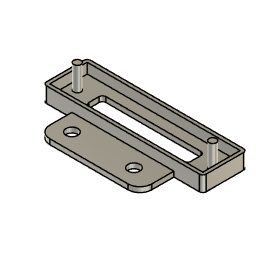
powerdist_ground_mount v2 (Autodesk Fusion 360 design; units mm, degrees)
Autodesk Fusion 360 part; units mm, degrees
sketch "Sketch1" plane through (0, 0, 0) normal (0, 0, 1) x (1, 0, 0)
  line L0 (0, 0) -> (94, 0)
  line L1 (94, 0) -> (94, 26)
  line L2 (94, 26) -> (0, 26)
  line L3 (0, 26) -> (0, 0)
  dimension "d1" = 94
  dimension "d2" = 26
  constraint horizontal L0
  constraint vertical L1
  constraint horizontal L2
  constraint vertical L3
  constraint coincident L0.start L3.end
  measures "d1" distance of L0.start L0.end
  measures "d2" distance of L0.start L2.end
extrude "Extrude1" add sketch "Sketch1" along normal blind 3
extrude "Extrude2" add 1 faces at (31.3333, 17.3333, 3) along direction (0, 0, 1) blind 6 thin wall 2 inside
sketch "Sketch2" plane through (0, 0, 3) normal (0, 0, 1) x (-1, 0, 0)
  line L0 (-92, -24) -> (-2, -24)
  line L1 (-2, -24) -> (-2, -2)
  line L2 (-2, -2) -> (-92, -2)
  line L3 (-92, -2) -> (-92, -24)
  circle A0 centre (-7.15, -13) radius 2.15
  circle A1 centre (-86.85, -13) radius 2.15
  dimension "d8" = 4.3
  dimension "d9" = 4.3
  dimension "d10" = 5.15
  dimension "d11" = 11
  dimension "d12" = 11
  dimension "d13" = 5.15
  measures "d8" diameter of A0
  measures "d9" diameter of A1
  measures "d10" distance of L1 A0.centre
  measures "d11" distance of L2 A0.centre
  measures "d12" distance of L2 A1.centre
  measures "d13" distance of L3 A1.centre
extrude "Extrude3" add sketch "Sketch2" along normal blind 14 contours A0 | A1
fillet "Fillet1" radius 2 4 edges at (94, 0, 4.5) (94, 26, 4.5) (0, 26, 4.5) (0, 0, 4.5)
sketch "Sketch3" plane through (0, 0, 9) normal (0, 0, 1) x (-1, 0, 0)
  line L0 (-2, -24) -> (-92, -24)
  line L1 (-92, -24) -> (-92, -2)
  line L2 (-92, -2) -> (-2, -2)
  line L3 (-2, -2) -> (-2, -24)
  arc A0 (0, -2) -> (-2, 0) centre (-2, -2) ccw
  line L4 (-2, 0) -> (-92, 0)
  arc A1 (-92, 0) -> (-94, -2) centre (-92, -2) ccw
  line L5 (-94, -2) -> (-94, -24)
  arc A2 (-94, -24) -> (-92, -26) centre (-92, -24) ccw
  line L6 (-92, -26) -> (-2, -26)
  arc A3 (-2, -26) -> (0, -24) centre (-2, -24) ccw
  line L7 (0, -24) -> (0, -2)
  line L8 (-77, 13) -> (-77, 0)
  arc A4 (-70, 20) -> (-77, 13) centre (-70, 13) ccw
  circle A5 centre (-63.5, 10) radius 3.5
  line L9 (-24, 20) -> (-70, 20)
  line L10 (-77, 0) -> (-17, 0)
  line L11 (-17, 0) -> (-17, 13)
  circle A6 centre (-27, 10) radius 3.5
  line L12 (-10.5, 0) -> (-76.5, 0)
  arc A7 (-17, 13) -> (-24, 20) centre (-24, 13) ccw
  point P0 (-43.5, 0)
  point P1 (-17, 20)
  dimension "d18" = 20
  dimension "d19" = 60
  dimension "d20" = 7
  dimension "d21" = 7
  dimension "d22" = 10
  dimension "d23" = 7
  constraint coincident L10.end L12
  constraint coincident P1 L11
  constraint coincident P1 L9
  constraint tangent L11 A7
  constraint tangent L9 A7
  constraint tangent A4 L9
  constraint tangent L8 A4
  constraint equal A4 A7
  constraint midpoint L4 L10
  measures "d18" distance of L10.end P1
  measures "d19" distance of L10.end L8.end
  measures "d20" diameter of A6
  measures "d21" diameter of A5
  measures "d22" distance of A6.centre L9
  measures "d23" radius of A7
extrude "Extrude4" add sketch "Sketch3" against normal blind 9 contours L4 L8 A4 L9 L10 L11 L12 A7
sketch "Sketch4" plane through (0, 0, 9) normal (0, 0, 1) x (-1, 0, 0)
  circle A0 centre (-63.5, 10) radius 3.5
  circle A1 centre (-27, 10) radius 3.5
  line L0 (-2, -24) -> (-92, -24)
  line L1 (-92, -24) -> (-92, -2)
  line L2 (-92, -2) -> (-2, -2)
  line L3 (-2, -2) -> (-2, -24)
  arc A2 (0, -2) -> (-2, 0) centre (-2, -2) ccw
  line L4 (-2, 0) -> (-17, 0)
  line L5 (-17, 0) -> (-17, 13)
  arc A3 (-17, 13) -> (-24, 20) centre (-24, 13) ccw
  line L6 (-24, 20) -> (-70, 20)
  arc A4 (-70, 20) -> (-77, 13) centre (-70, 13) ccw
  line L7 (-77, 13) -> (-77, 0)
  line L8 (-77, 0) -> (-92, 0)
  arc A5 (-92, 0) -> (-94, -2) centre (-92, -2) ccw
  line L9 (-94, -2) -> (-94, -24)
  arc A6 (-94, -24) -> (-92, -26) centre (-92, -24) ccw
  line L10 (-92, -26) -> (-2, -26)
  arc A7 (-2, -26) -> (0, -24) centre (-2, -24) ccw
  line L11 (0, -24) -> (0, -2)
  line L12 (-77, 0) -> (-17, 0)
  constraint coincident L7.end L8.start
  constraint coincident L4.end L5.start
extrude "Extrude5" cut sketch "Sketch4" against normal blind 6 contours L5 A3 L6 A4 L7 L12
sketch "Sketch5" plane through (0, 0, 3) normal (0, 0, 1) x (-1, 0, 0)
  circle A0 centre (-86.85, -13) radius 2.15
  circle A1 centre (-7.15, -13) radius 2.15
  line L0 (-92, -24) -> (-2, -24)
  line L1 (-2, -24) -> (-2, -2)
  line L2 (-2, -2) -> (-92, -2)
  line L3 (-92, -2) -> (-92, -24)
  line L4 (-19, -18) -> (-75, -18)
  line L5 (-77, -16) -> (-77, -10)
  line L6 (-75, -8) -> (-19, -8)
  line L7 (-17, -10) -> (-17, -16)
  arc A2 (-19, -18) -> (-17, -16) centre (-19, -16) ccw
  arc A3 (-77, -16) -> (-75, -18) centre (-75, -16) ccw
  arc A4 (-75, -8) -> (-77, -10) centre (-75, -10) ccw
  arc A5 (-17, -10) -> (-19, -8) centre (-19, -10) ccw
  point P0 (-17, -18)
  point P1 (-77, -18)
  point P2 (-17, -8)
  dimension "d28" = 60
  dimension "d29" = 10
  dimension "d30" = 6
  dimension "d31" = 15
  dimension "d32" = 2
  constraint horizontal L4
  constraint vertical L5
  constraint horizontal L6
  constraint vertical L7
  constraint coincident P0 L4
  constraint coincident P0 L7
  constraint tangent L4 A2
  constraint tangent L7 A2
  constraint coincident P1 L4
  constraint coincident P1 L5
  constraint tangent L4 A3
  constraint tangent L5 A3
  constraint equal A2 A3
  constraint tangent L5 A4
  constraint tangent L6 A4
  constraint equal A2 A4
  constraint coincident P2 L6
  constraint coincident P2 L7
  constraint tangent L6 A5
  constraint tangent L7 A5
  constraint equal A2 A5
  measures "d28" distance of P0 P1
  measures "d29" distance of P0 P2
  measures "d30" distance of L0 L4
  measures "d31" distance of L1 L7
  measures "d32" radius of A2
extrude "Extrude6" cut sketch "Sketch5" against normal blind 3 contours L4 L5 L6 L7 A2 A3 A4 A5
